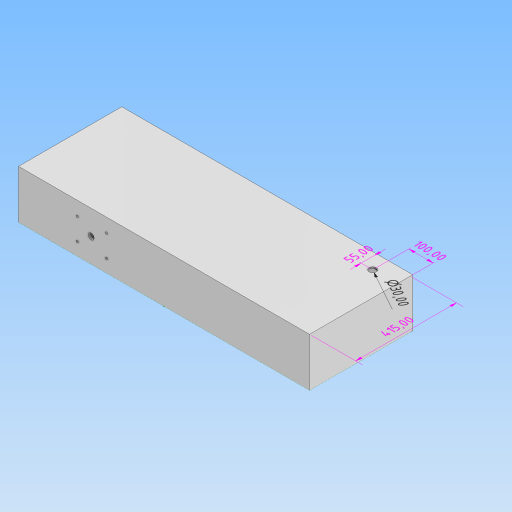
# Autodesk Inventor part: Mittelkonsole
Saved by Autodesk Inventor 2024.4 (Build 284460000, 460)
## iProperties
Created: 2026-01-19
Part Number: Mittelkonsole
Material: Generisch
Document SubType Name: Modeling
Designer: windows-desktop
Density: 1 g/cm^3
Appearance: Vorgabe
Mass: 16002.9 g
Surface Area: 37309.3 cm^2
Volume: 16002.9 cm^3
Masse[kg]: 16,0 kg
Autodesk Inventor part; units mm, degrees
ref_plane "YZ Plane" through (0, 0, 0) normal (1, 0, 0) x (0, 1, 0)
ref_plane "XZ Plane" through (0, 0, 0) normal (0, 1, 0) x (-1, 0, 0)
sketch "Skizze1" plane through (0, 0, 0) normal (0, 1, 0) x (-1, 0, 0)
  line L0 (599, 100) -> (-599, 100)
  line L1 (-599, 100) -> (-599, -100)
  line L2 (-599, -100) -> (599, -100)
  line L3 (599, -100) -> (599, 100)
  line L4 (838.6, 0) -> (-838.6, 0) construction
  line L5 (0, -140) -> (0, 140) construction
  point P0 (0, 0)
  dimension "d0" = 1198
  dimension "d1" = 200
  constraints: 8 end point, 2 parallel, 1 horizontal, 1 perpendicular, 2 other
  measures "d0" distance of L2.end L1.end
  measures "d1" distance of L1.end L0.end
extrude "Extrusion1" add sketch "Skizze1" along normal blind 420
shell "Wandung1" thickness 5 removed faces 1 at (199.6667, 0, -33.3333)
sketch "Skizze2" plane through (-599, 0, 100) normal (0, 0, 1) x (1, 0, 0)
  line L0 (0, 0) -> (1198, 0) construction
  line L1 (1198, 0) -> (1098, 0)
  line L2 (1098, 0) -> (1098, 130)
  line L3 (1098, 130) -> (1098, 360)
  point P0 (599, 0)
  dimension "d9" = 100
  dimension "d10" = 130
  dimension "d11" = 230
  constraints: 6 end point, 1 perpendicular, 1 point on line, 1 vertical
  measures "d9" distance of L0.end L1.end
  measures "d10" distance of L1.end L2.end
  measures "d11" distance of L2.end L3.end
hole "Bohrung1" at (499, 360, 100) direction (0, 0, -1) diameter 30 depth 20 tip angle 118
ref_plane "Arbeitsebene1" through (0, 310.83, 0) normal (0, 1, 0) x (1, 0, 0)
sketch "Skizze3" plane through (0, 310.83, 0) normal (0, 1, 0) x (1, 0, 0)
  line L0 (599, 100) -> (-599, 100) construction
  line L1 (599, -100) -> (599, 100) construction
  line L2 (-599, -100) -> (599, -100) construction
  line L3 (-599, 100) -> (-599, -100) construction
  line L4 (599, -100) -> (499, -100)
  line L5 (499, -100) -> (511.5, -100)
  line L6 (499, -100) -> (486.5, -100)
  line L7 (-599, 100) -> (599, 100)
  line L8 (599, 100) -> (599, -100)
  line L9 (599, -100) -> (-599, -100)
  line L10 (-599, -100) -> (-599, 100)
  line L11 (599, 0) -> (86.8278, 0)
  line L12 (499, -100) -> (499, 0)
  line L13 (499, 0) -> (499, 100)
  line L14 (499, 0) -> (536.585, 0)
  line L15 (499, 0) -> (463.415, 0)
  line L16 (499, 0) -> (464.19, 0)
  line L17 (499, 0) -> (499, 36.585)
  line L18 (499, 36.585) -> (535.585, 36.585)
  line L19 (535.585, 36.585) -> (441.933, 36.585)
  line L20 (441.933, 36.585) -> (441.933, -36.585)
  line L21 (441.933, -36.585) -> (535.585, -36.585)
  line L22 (535.585, -36.585) -> (535.585, -71.395)
  line L23 (535.585, -71.395) -> (441.933, -71.395)
  line L24 (441.933, -71.395) -> (407.123, -71.395)
  line L25 (407.123, -71.395) -> (407.123, 36.585)
  line L26 (407.123, 36.585) -> (407.123, 71.395)
  line L27 (407.123, 71.395) -> (535.585, 71.395)
  line L28 (535.585, 71.395) -> (535.585, 36.585)
  point P0 (0, 0)
  dimension "d20" = 100
  dimension "d21" = 12.5
  dimension "d22" = 12.5
  dimension "d33" = 36.585
  dimension "d34" = 36.585
  dimension "d35" = 93.652
  dimension "d36" = 73.17
  dimension "d37" = 93.652
  dimension "d38" = 34.81
  dimension "d39" = 34.81
  dimension "d40" = 34.81
  constraints: 50 end point, 13 point on line, 8 perpendicular, 2 horizontal, 2 parallel, 1 midpoint, 1 vertical
  measures "d20" distance of L1.start L4.end
  measures "d21" distance of L4.end L5.end
  measures "d22" distance of L4.end L6.end
  measures "d33" distance of L12.end L17.end
  measures "d34" distance of L17.end L18.end
  measures "d35" distance of L18.end L19.end
  measures "d36" distance of L19.end L20.end
  measures "d37" distance of L20.end L21.end
  measures "d38" distance of L21.end L22.end
  measures "d39" distance of L23.end L24.end
  measures "d40" distance of L25.end L26.end
extrude "Extrusion2" add sketch "Skizze3" against normal blind 20
sketch "Skizze6" plane through (-599, 0, 100) normal (0, 0, 1) x (1, 0, 0)
  circle A0 centre (1098, 360) radius 15 construction
  line L0 (5, 310.83) -> (1193, 310.83) construction
  arc A1 (1113, 360) -> (1083, 360) centre (1098, 360) ccw
  line L1 (1083, 360) -> (1083, 310.83)
  line L2 (1113, 360) -> (1113, 310.83)
  circle A2 centre (1098, 360) radius 15
  point P0 (599, 0)
  dimension "d25" = 30
  constraints: 4 end point, 2 centre point, 2 coincident, 2 perpendicular, 2 point on circle, 2 point on line, 2 tangent, 1 concentric
  measures "d25" diameter of A1
extrude "Extrusion3" add sketch "Skizze3" along normal blind 85 contours L23 L24 L25 L11 L20 L21 L12 | L12 L21 L22 L23 | L27 L28 L18 L13 | L13 L19 L20 L11 L25 L26 L27
ref_plane "Arbeitsebene2" through (0, 360, 0) normal (0, 1, 0) x (1, 0, 0)
sketch "Skizze7" plane through (0, 0, 0) normal (0, 0, 1) x (1, 0, 0)
  circle A0 centre (499, 360) radius 15 construction
  circle A1 centre (499, 360) radius 32
  circle A2 centre (499, 360) radius 32
  point P0 (0, 0)
  dimension "d44" = 64
  constraints: 2 centre point, 2 coincident, 1 concentric
  measures "d44" diameter of A1
extrude "Extrusion4" cut sketch "Skizze7" along normal mid plane 107.17
sketch "Skizze8" plane through (0, 420, 0) normal (0, 1, 0) x (1, 0, 0)
  line L0 (-599, 100) -> (599, 100)
  line L1 (599, 100) -> (599, -100)
  line L2 (599, -100) -> (-599, -100)
  line L3 (-599, -100) -> (-599, 100)
  point P0 (0, 0)
  constraints: 8 end point, 2 parallel, 1 horizontal, 1 perpendicular
extrude "Extrusion5" cut sketch "Skizze8" against normal blind 5
hole "Bohrung2" at (499, 360, 100) direction (0, 0, -1) diameter 20 depth 500 tip angle 118
sketch "Skizze9" plane through (441.933, 310.83, -36.585) normal (1, 0, 0) x (0, 0, -1)
  line L0 (0, 0) -> (0, 85) construction
  line L1 (-73.17, 85) -> (0, 85) construction
  line L2 (-73.17, 0) -> (-73.17, 85) construction
  line L3 (-73.17, 85) -> (0, 85)
  line L4 (-73.17, 85) -> (-73.17, 0)
  line L5 (0, 0) -> (-73.17, 0)
  line L6 (-107.98, 0) -> (34.81, 0) construction
  line L7 (0, 0) -> (0, 85)
  line L8 (-36.585, 0) -> (-36.585, 49.17)
  circle A0 centre (-36.585, 49.17) radius 32
  circle A1 centre (-36.585, 49.17) radius 17.5
  point P0 (-36.585, -310.83)
  dimension "d56" = 49.17
  dimension "d58" = 64
  dimension "d61" = 35
  constraints: 10 end point, 4 collinear, 2 centre point, 2 coincident, 1 midpoint, 1 vertical
  measures "d56" distance of L8.start L8.end
  measures "d58" diameter of A0
  measures "d61" diameter of A1
extrude "Extrusion6" cut sketch "Skizze9" against normal blind 5 contours A1 | A0
extrude "Extrusion7" cut sketch "Skizze9" against normal blind 50 contours A1
sketch "Skizze10" plane through (0, 310.83, 0) normal (0, 1, 0) x (1, 0, 0)
  line L0 (-600.9138, 0) -> (-300.0038, 0)
  circle A0 centre (-300.0038, 0) radius 17.5
  line L1 (-300.0038, 0) -> (-206.3518, 0)
  line L2 (-262.3958, 0) -> (-262.3958, 70)
  line L3 (-262.3958, 70) -> (-232.3958, 70)
  line L4 (-232.3958, 70) -> (-232.3958, -70)
  line L5 (-232.3958, -70) -> (-262.3958, -70)
  line L6 (-262.3958, -70) -> (-262.3958, 0)
  line L7 (-300.0038, 0) -> (-263.4188, 0)
  line L8 (-300.0038, 0) -> (-262.3958, 0)
  point P0 (0, 0)
  dimension "d64" = 300.91
  dimension "d72" = 35
  dimension "d74" = 93.652
  dimension "d75" = 70
  dimension "d76" = 30
  dimension "d77" = 140
  dimension "d86" = 36.585
  dimension "d87" = 37.608
  constraints: 18 end point, 3 horizontal, 3 perpendicular, 2 point on line, 1 centre point, 1 coincident, 1 vertical
  measures "d64" distance of L0.start L0.end
  measures "d72" diameter of A0
  measures "d74" distance of L1.end L1.start
  measures "d75" distance of L2.start L2.end
  measures "d76" distance of L2.end L3.end
  measures "d77" distance of L3.end L4.end
  measures "d86" distance of L1.start L7.end
  measures "d87" distance of L1.start L8.end
hole "Bohrung3" at (-300.0038, 310.83, 0) direction (0, -1, 0) diameter 64 depth 500 tip angle 118
extrude "Extrusion8" add sketch "Skizze10" along normal blind 104.17 contours L2 L3 L4 L1 | L1 L4 L5 L6
sketch "Skizze11" plane through (-262.3958, 310.83, -70) normal (-1, 0, 0) x (0, 0, 1)
  line L0 (-70, 49.17) -> (210, 49.17) construction
  circle A0 centre (70, 49.17) radius 17.5 construction
  circle A1 centre (70, 49.17) radius 32
  circle A2 centre (70, 49.17) radius 17.75
  point P0 (70, -310.83)
  dimension "d80" = 64
  dimension "d83" = 35.5
  constraints: 2 centre point, 2 coincident
  measures "d80" diameter of A1
  measures "d83" diameter of A2
extrude "Extrusion9" cut sketch "Skizze11" against normal blind 12 contours A1 | A2
extrude "Extrusion10" cut sketch "Skizze11" against normal blind 40 contours A2
sketch "Skizze12" plane through (0, 310.83, 0) normal (0, 1, 0) x (1, 0, 0)
  circle A0 centre (-300.0038, 0) radius 32 construction
  circle A1 centre (-300.0038, 0) radius 40
  circle A2 centre (-300.0038, 0) radius 32
  point P0 (0, 0)
  dimension "d88" = 80
  constraints: 2 centre point, 2 coincident, 1 concentric
  measures "d88" diameter of A1
extrude "Extrusion11" add sketch "Skizze12" against normal blind 4
sketch "Skizze13" plane through (0, 0, 0) normal (0, -1, 0) x (1, 0, 0)
  circle A0 centre (-300.0038, 0) radius 32 construction
  circle A1 centre (-300.0038, 0) radius 12.5
  line L0 (-268.0493, -31.9545) -> (-331.9583, 31.9545) construction
  line L1 (-331.9583, -31.9545) -> (-268.0493, 31.9545) construction
  line L2 (-594, 95) -> (594, 95)
  line L3 (594, 95) -> (594, -95)
  line L4 (594, -95) -> (-594, -95)
  line L5 (-594, -95) -> (-594, 95)
  point P0 (0, 0)
  dimension "d101" = 25
  constraints: 12 end point, 2 midpoint, 2 parallel, 1 centre point, 1 coincident, 1 horizontal, 1 perpendicular
  measures "d101" diameter of A1
extrude "Extrusion12" add sketch "Skizze13" against normal blind 10
sketch "Skizze14" plane through (599, 0, -100) normal (0, 0, -1) x (-1, 0, 0)
  circle A0 centre (100, 360) radius 10 construction
  circle A1 centre (100, 360) radius 15
  point P0 (599, 0)
  dimension "d104" = 30
  constraints: 1 centre point, 1 coincident
  measures "d104" diameter of A1
hole "Bohrung4" at (499, 360, -100) direction (0, 0, 1) diameter 30 depth 20 tip angle 118
sketch "Skizze16" plane through (-232.3958, 310.83, 70) normal (1, 0, 0) x (0, 0, -1)
  circle A0 centre (70, 49.17) radius 17.75 construction
  circle A1 centre (70, 49.17) radius 23.5
  point P0 (70, -310.83)
  dimension "d112" = 47
  constraints: 1 centre point, 1 coincident
  measures "d112" diameter of A1
extrude "Extrusion13" cut sketch "Skizze16" against normal blind 6.4
sketch "Skizze17" plane through (407.123, 310.83, 71.395) normal (-1, 0, 0) x (0, 0, 1)
  circle A0 centre (-71.395, 49.17) radius 17.5 construction
  circle A1 centre (-71.395, 49.17) radius 23.5
  point P0 (-71.395, -310.83)
  dimension "d115" = 47
  constraints: 1 centre point, 1 coincident
  measures "d115" diameter of A1
extrude "Extrusion14" cut sketch "Skizze17" against normal blind 6.4
sketch "Skizze18" plane through (407.123, 310.83, 71.395) normal (0, 0, 1) x (1, 0, 0)
  circle A0 centre (91.877, 49.17) radius 10 construction
  circle A1 centre (91.877, 49.17) radius 16
  point P0 (-407.123, -310.83)
  dimension "d118" = 32
  constraints: 1 centre point, 1 coincident
  measures "d118" diameter of A1
extrude "Extrusion15" cut sketch "Skizze18" against normal blind 7
sketch "Skizze19" plane through (535.585, 310.83, -71.395) normal (0, 0, -1) x (-1, 0, 0)
  circle A0 centre (36.585, 49.17) radius 16 construction
  circle A1 centre (36.585, 49.17) radius 16
  point P0 (535.585, -310.83)
  dimension "d121" = 32
  constraints: 1 centre point, 1 coincident
  measures "d121" diameter of A1
extrude "Extrusion16" cut sketch "Skizze19" against normal blind 7
sketch "Skizze20" plane through (0, 310.83, 0) normal (0, 1, 0) x (1, 0, 0)
  circle A0 centre (-300.0038, 0) radius 32 construction
  circle A1 centre (-300.0038, 0) radius 40
  point P0 (0, 0)
  dimension "d124" = 80
  constraints: 1 centre point, 1 coincident
  measures "d124" diameter of A1
extrude "Extrusion17" cut sketch "Skizze20" against normal blind 12
sketch "Skizze21" plane through (599, 0, -100) normal (0, 0, -1) x (-1, 0, 0)
  circle A0 centre (100, 360) radius 15 construction
  line L0 (1198, 415) -> (0, 415) construction
  line L1 (0, 0) -> (0, 415) construction
  line L2 (0, 0) -> (1198, 0) construction
  line L3 (1198, 0) -> (1198, 415) construction
  point P0 (599, 0)
sketch "Skizze22" plane through (0, 0, 0) normal (0, -1, 0) x (1, 0, 0)
  circle A0 centre (-356.8903, 42.7877) radius 5.0941 construction
  circle A1 centre (-298.864, 3.8435) radius 17.5 construction
  circle A2 centre (-298.864, 3.8435) radius 17.5 construction
  point P0 (0, 0)
  point P1 (-236.8903, 42.7877)
  point P2 (-236.8903, -47.2123)
  point P3 (-356.8903, -47.2123)
  point P4 (-236.8903, 42.7877)
  point P5 (-236.8903, -47.2123)
  point P6 (-356.8903, -47.2123)
  constraints: 5 coincident, 3 centre point, 1 concentric
hole "Bohrung5" at (-356.8903, 0, 42.7877) at (-236.8903, 0, 42.7877) at (-236.8903, 0, -47.2123) at (-356.8903, 0, -47.2123) direction (0, 1, 0) diameter 9.3762 depth 29.3 tip angle 118 thread size "M11x1.5" class "6H" standard "ISO Metric profile"
sketch "Skizze23" plane through (0, 415, 0) normal (0, 1, 0) x (1, 0, 0)
  line L0 (-599, 100) -> (599, 100)
  line L1 (599, 100) -> (599, -100)
  line L2 (599, -100) -> (-599, -100)
  line L3 (-599, -100) -> (-599, 100)
  point P0 (0, 0)
  constraints: 8 end point, 2 parallel, 1 horizontal, 1 perpendicular
extrude "Extrusion18" add sketch "Skizze23" along normal blind 10
